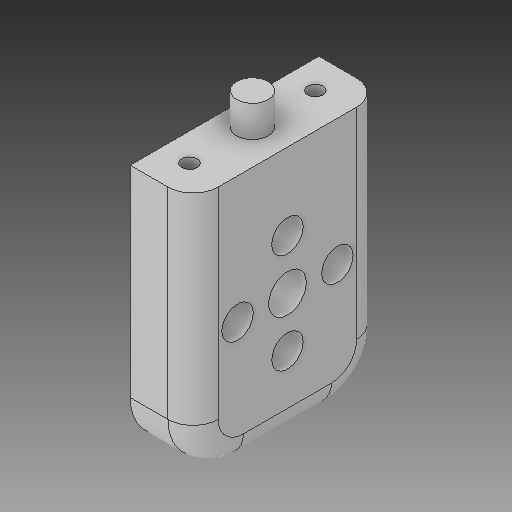
# Autodesk Inventor part: TapaPieEfector
Saved by Autodesk Inventor 2019 (Build 230136000, 136)
## iProperties
Created: 2016-12-20
Part Number: TapaPieEfector
Material: Genérico
Document SubType Name: Modeling
Designer: Mario
Density: 1 g/cm^3
Appearance: Por defecto
Author: Mario
Autodesk Inventor part; units mm, degrees
ref_plane "YZ Plane" through (0, 0, 0) normal (1, 0, 0) x (0, 1, 0)
ref_plane "XZ Plane" through (0, 0, 0) normal (0, 1, 0) x (-1, 0, 0)
ref_plane "XY Plane" through (0, 0, 0) normal (0, 0, 1) x (1, 0, 0)
sketch "Sketch1" plane through (0, 0, 0) normal (1, 0, 0) x (0, 1, 0)
  line L0 (15, 15) -> (-15, 15)
  line L1 (-15, -15) -> (15, -15)
  line L2 (15, -15) -> (15, 15)
  line L3 (15, 15) -> (-15, -15) construction
  line L4 (-15, 15) -> (15, -15) construction
  line L5 (-15, -15) -> (-25, -15)
  line L6 (-25, -15) -> (-25, 15)
  line L7 (-25, 15) -> (-15, 15)
  point P0 (0, 0)
  dimension "d0" = 30
  dimension "d1" = 30
  dimension "d13" = 10
  constraints: 16 end point, 2 horizontal, 2 midpoint, 2 perpendicular, 1 parallel
  measures "d0" distance of L1.end L1.start
  measures "d1" distance of L1.start L0.end
  measures "d13" distance of L1.start L5.end
extrude "Extrusion1" add sketch "Sketch1" along normal blind 10
sketch "Sketch2" plane through (0, 0, 0) normal (-1, 0, 0) x (0, 0, 1)
  line L0 (-13, -13) -> (-13, 13)
  line L1 (13, 13) -> (13, -13)
  line L2 (13, 13) -> (-13, 13)
  line L3 (-13, -13) -> (-13, -23)
  line L4 (-13, -23) -> (13, -23)
  line L5 (13, -23) -> (13, -13)
  point P0 (0, 0)
  dimension "d14" = 10
  constraints: 12 end point, 1 perpendicular, 1 vertical
  measures "d14" distance of L0.start L3.end
extrude "Extrusion2" cut sketch "Sketch2" against normal blind 8
sketch "Sketch3" plane through (0, 15, 15) normal (0, 1, 0) x (1, 0, 0)
  circle A0 centre (4.4342, 15) radius 2.5 projected
  point P0 (0, 15)
extrude "Extrusion3" add sketch "Sketch3" along normal blind 5
sketch "Sketch4" plane through (0, 13, -13) normal (0, -1, 0) x (1, 0, 0)
  circle A0 centre (4.4342, 23) radius 1.225 projected
  circle A1 centre (4.4342, 3) radius 1.225 projected
  point P0 (0, 13)
extrude "Extrusion4" cut sketch "Sketch4" against normal blind 2
fillet "Fillet4" radius 8 4 edges at (4, -23, 13) (4, -23, -13) (5, -25, -15) (5, -25, 15)
fillet "Fillet5" radius 4 4 edges at (10, -25, 0) (10, -22.6569, 12.6569) (10, -1, -15) (10, -22.6569, -12.6569)
sketch "Sketch5" plane through (8, 0, 0) normal (-1, 0, 0) x (0, 0, 1)
  arc A0 (12.525, -5.1293) -> (-12.525, -5.1293) centre (0, -5.1293) ccw
  circle A1 centre (0, -5.1293) radius 11.025
  arc A2 (5, -23) -> (13, -15) centre (5, -15) ccw
  line L0 (13, -5.1293) -> (13, -15)
  line L1 (5, -23) -> (-5, -23)
  arc A3 (-13, -15) -> (-5, -23) centre (-5, -15) ccw
  line L2 (-13, -15) -> (-13, -5.1293)
  line L3 (12.525, -5.1293) -> (13, -5.1293)
  line L4 (13, -5.1293) -> (13, -15)
  line L5 (-12.525, -5.1293) -> (-13, -5.1293)
  line L6 (-13, -15) -> (-13, -5.1293)
  point P0 (0, 0)
  constraints: 14 end point, 6 point on circle, 4 centre point, 2 point on line
extrude "Extrusion5" add sketch "Sketch5" along normal blind 8
sketch "Sketch6" plane through (8, -5.1293, 0) normal (-1, 0, 0) x (0, 0, 1)
  circle A0 centre (0, 0) radius 11.025 projected
  point P0 (0, 5.1293)
extrude "Extrusion6" add sketch "Sketch6" along normal blind 4.5
sketch "Sketch7" plane through (10, 0, 0) normal (1, 0, 0) x (0, 0, -1)
  circle A0 centre (0, -5.1293) radius 1.525
  point P0 (0, 0)
  constraints: 1 centre point
extrude "Extrusion7" cut sketch "Sketch7" against normal blind 8
sketch "Sketch8" plane through (10, 0, 0) normal (1, 0, 0) x (0, 0, -1)
  circle A0 centre (0, -5.1293) radius 1.525 projected
  circle A1 centre (0, -5.1293) radius 3
  point P0 (0, 0)
  dimension "d29" = 6
  constraints: 1 centre point, 1 coincident
  measures "d29" diameter of A1
extrude "Extrusion8" cut sketch "Sketch8" against normal blind 5
sketch "Sketch9" plane through (10, 0, 0) normal (1, 0, 0) x (0, 0, -1)
  circle A0 centre (0, -5.1293) radius 11.025 projected
  line L0 (0, -5.1293) -> (0, -13.0693)
  line L1 (0, -5.1293) -> (0, 2.8107)
  circle A1 centre (0, -5.1293) radius 1.525 projected
  line L2 (0, -5.1293) -> (7.94, -5.1293)
  line L3 (0, -5.1293) -> (-7.94, -5.1293)
  circle A2 centre (7.94, -5.1293) radius 1.59
  circle A3 centre (0, -13.0693) radius 1.59
  circle A4 centre (-7.94, -5.1293) radius 1.59
  circle A5 centre (0, 2.8107) radius 1.59
  point P0 (0, 0)
  dimension "d32" = 7.94
  dimension "d33" = 7.94
  dimension "d34" = 7.94
  dimension "d35" = 7.94
  dimension "d36" = 3.18
  dimension "d37" = 3.18
  dimension "d38" = 3.18
  dimension "d39" = 3.18
  constraints: 8 end point, 4 centre point, 2 horizontal, 2 vertical, 1 coincident
  measures "d32" distance of L0.start L0.end
  measures "d33" distance of L0.start L1.end
  measures "d34" distance of L2.start L2.end
  measures "d35" distance of L2.start L3.end
  measures "d36" diameter of A2
  measures "d37" diameter of A3
  measures "d38" diameter of A4
  measures "d39" diameter of A5
extrude "Extrusion9" cut sketch "Sketch9" against normal blind 8 contours A3 | A4 | A5 | A2
sketch "Sketch10" plane through (10, 0, 0) normal (1, 0, 0) x (0, 0, -1)
  circle A0 centre (0, 2.8107) radius 1.59 projected
  circle A1 centre (7.94, -5.1293) radius 1.59 projected
  circle A2 centre (0, -13.0693) radius 1.59 projected
  circle A3 centre (-7.94, -5.1293) radius 1.59 projected
  circle A4 centre (0, 2.8107) radius 2.5
  circle A5 centre (7.94, -5.1293) radius 2.5
  circle A6 centre (0, -13.0693) radius 2.5
  circle A7 centre (-7.94, -5.1293) radius 2.5
  point P0 (0, 0)
  dimension "d42" = 5
  dimension "d43" = 5
  dimension "d44" = 5
  dimension "d45" = 5
  constraints: 4 centre point, 1 coincident
  measures "d42" diameter of A4
  measures "d43" diameter of A5
  measures "d44" diameter of A6
  measures "d45" diameter of A7
extrude "Extrusion10" cut sketch "Sketch10" against normal blind 5
body "Solid1"
